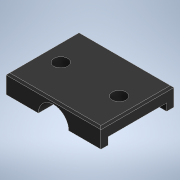
# Autodesk Inventor part: BottomAcrylicSheetRodHolder_1
Saved by Autodesk Inventor 2021 (Build 250183000, 183)
## iProperties
Created: 2020-07-16
Part Number: BottomAcrylicSheetRodHolder_1
Material: Generic
Document SubType Name: Modeling
Designer: CASE-SMALL2
Density: 1 g/cm^3
Appearance: Default
Author: CASE-SMALL2
## iProperties of the stored document _3DPrint.ipt
Created: 2020-07-17
Part Number: _3DPrint
Material: Generic
Document SubType Name: Modeling
Designer: CASE-SMALL2
Density: 1 g/cm^3
Appearance: Default
Author: CASE-SMALL2
Autodesk Inventor part; units mm, degrees
ref_plane "YZ Plane" through (0, 0, 0) normal (1, 0, 0) x (0, 1, 0)
ref_plane "XZ Plane" through (0, 0, 0) normal (0, 1, 0) x (-1, 0, 0)
ref_plane "XY Plane" through (0, 0, 0) normal (0, 0, 1) x (1, 0, 0)
sketch "Sketch1" plane through (0, 0, 0) normal (0, 0, 1) x (1, 0, 0)
  arc A0 (4.15, 0) -> (-4.15, 0) centre (0, 0) ccw
  line L0 (-21.6509, 0) -> (19.2313, 0) projected
  line L1 (-13, 0) -> (-13, 5.15)
  line L2 (-13, 5.15) -> (13, 5.15)
  line L3 (13, 5.15) -> (13, 0)
  line L4 (-13, 0) -> (-4.15, 0)
  line L5 (4.15, 0) -> (13, 0)
  dimension "d0" = 8.3
  dimension "d1" = 1
  dimension "d2" = 13
  dimension "d3" = 13
  constraints: 10 end point, 4 point on line, 2 perpendicular, 2 point on circle, 1 centre point, 1 coincident, 1 collinear, 1 vertical
  measures "d0" diameter of A0
  measures "d1" distance edge to line of A0 L2
  measures "d2" distance from line of point (0, 0) L3
  measures "d3" distance from line of point (0, 0) L1
extrude "Extrusion1" add sketch "Sketch1" along normal blind 20 contours A0 L0 L1 L2 L3
sketch "Sketch2" plane through (-13, 5.15, 0) normal (0, 1, 0) x (1, 0, 0)
  line L0 (-4.8106, -10) -> (24.391, -10) construction
  line L1 (26, 0) -> (0, 0) construction
  line L2 (26, -20) -> (0, -20) construction
  circle A0 centre (5, -10) radius 1.9
  circle A1 centre (21, -10) radius 1.9
  point P0 (13, 0)
  dimension "d7" = 20
  dimension "d8" = 10
  dimension "d9" = 3.8
  dimension "d10" = 3.8
  dimension "d11" = 16
  dimension "d12" = 8
  constraints: 2 centre point, 2 end point, 2 point on line, 1 horizontal
  measures "d7" distance between parallel lines of L1 L2
  measures "d8" distance between parallel lines of L0 L2
  measures "d9" diameter of A0
  measures "d10" diameter of A1
  measures "d11" distance of A1.centre A0.centre
  measures "d12" horizontal distance of point (13, 0) A0.centre
extrude "Extrusion2" cut sketch "Sketch2" against normal through all
sketch "Sketch3" plane through (-13, 0, 0) normal (0, -1, 0) x (1, 0, 0)
  line L0 (0, 0) -> (0, 20) projected
  line L1 (0, 2) -> (2, 2)
  line L2 (2, 2) -> (2, 18)
  line L3 (2, 18) -> (0, 18)
  line L4 (0, 18) -> (0, 2)
  line L5 (26, 0) -> (26, 20) projected
  line L6 (26, 2) -> (24, 2)
  line L7 (24, 2) -> (24, 18)
  line L8 (24, 18) -> (26, 18)
  line L9 (26, 18) -> (26, 2)
  line L10 (0, 0) -> (8.85, 0) projected
  line L11 (0, 20) -> (8.85, 20) projected
  line L12 (17.15, 20) -> (26, 20) projected
  line L13 (17.15, 0) -> (26, 0) projected
  point P0 (13, 0)
  point P1 (0, 18)
  dimension "d15" = 2
  dimension "d16" = 2
  dimension "d17" = 2
  dimension "d18" = 2
  dimension "d19" = 2
  dimension "d20" = 2
  constraints: 16 end point, 4 parallel, 2 horizontal, 2 perpendicular, 2 point on line
  measures "d15" distance between parallel lines of L10 L1
  measures "d16" distance between parallel lines of L11 L3
  measures "d17" distance between parallel lines of L0 L2
  measures "d18" distance between parallel lines of L12 L8
  measures "d19" distance between parallel lines of L9 L7
  measures "d20" distance between parallel lines of L13 L6
extrude "Extrusion3" cut sketch "Sketch3" against normal blind 2
chamfer "Chamfer1" distance 0.5 angle 45 4 edges at (13, 5.15, 10) (0, 5.15, 20) (-13, 5.15, 10) (0, 5.15, 0)
equation "\"d3\" = d2"
equation "\"d8\" = 0.5 * d7"
equation "\"d10\" = d9"
equation "\"d16\" = d15"
equation "\"d17\" = d15"
equation "\"d18\" = d16"
equation "\"d19\" = d16"
equation "\"d20\" = d17"
body "Solid1"
